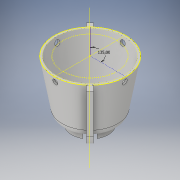
# Autodesk Inventor part: pot1
Saved by Autodesk Inventor 2019 (Build 230136000, 136)
## iProperties
Created: 2019-11-02
Part Number: pot1
Material: Generic
Document SubType Name: Modeling
Designer: assman
Density: 1 g/cm^3
Appearance: Default
Author: assman
## iProperties of the stored document pot1_3DPrint.ipt
Created: 2019-11-02
Part Number: pot1_3DPrint
Material: Generic
Document SubType Name: Modeling
Designer: assman
Density: 1 g/cm^3
Appearance: Default
Author: assman
Autodesk Inventor part; units mm, degrees
ref_plane "YZ Plane" through (0, 0, 0) normal (1, 0, 0) x (0, 1, 0)
ref_plane "XZ Plane" through (0, 0, 0) normal (0, 1, 0) x (-1, 0, 0)
ref_plane "XY Plane" through (0, 0, 0) normal (0, 0, 1) x (1, 0, 0)
sketch "Sketch2" plane through (0, 0, 0) normal (0, 0, 1) x (1, 0, 0)
  line L0 (0, 0) -> (28.321801, 0)
  line L1 (30.291416, 1.652704) -> (42.155372, 68.936543)
  arc A0 (28.321801, 0) -> (30.291416, 1.652704) centre (28.321801, 2) ccw
  line L2 (42.155372, 68.936543) -> (0, 68.936543)
  line L3 (0, 68.936543) -> (0, 0)
  point P0 (30, 0)
  dimension "d2" = 30
  dimension "d3" = 70
  dimension "d5" = 2
  constraints: 8 end point, 2 horizontal, 2 point on circle, 2 point on line, 2 tangent, 1 centre point, 1 perpendicular
  measures "d2" distance of L0.start point (30, 0)
  measures "d3" distance of point (30, 0) L1.end
  measures "d5" radius of A0
revolve "Revolution1" add sketch "Sketch2" angle 360 about axis through (0, 68.936543, 0) along (0, -1, 0)
sketch "Sketch3" plane through (0, 0, 0) normal (0, 0, 1) x (1, 0, 0)
  line L0 (42.155372, 68.936543) -> (30.291416, 1.652704)
  line L1 (-28.321801, 0) -> (28.321801, 0)
  arc A0 (28.321801, 0) -> (30.291416, 1.652704) centre (28.321801, 2) ccw
  line L2 (-28.321801, 0) -> (28.321801, 0)
  line L3 (33.488192, 70.4648) -> (21.624236, 3.180961)
  line L4 (0, -10) -> (28.321801, -10)
  line L5 (52.309639, 68.936543) -> (40.139494, -0.083778)
  arc A1 (28.321801, -10) -> (40.139494, -0.083778) centre (28.321801, 2) ccw
  line L6 (42.155372, 68.936543) -> (52.309639, 68.936543)
  line L7 (-42.155372, 68.936543) -> (42.155372, 68.936543)
  line L8 (0, 68.936543) -> (0, -10)
  line L9 (0, 68.936543) -> (42.155372, 68.936543)
  point P0 (0, 0)
  dimension "d7" = 10
  dimension "d8" = 10
  constraints: 14 end point, 3 parallel, 2 point on circle, 1 centre point, 1 collinear, 1 horizontal, 1 midpoint, 1 perpendicular, 1 tangent
  measures "d7" distance between parallel lines of L1 L4
  measures "d8" distance between parallel lines of L0 L5
revolve "Revolution2" add sketch "Sketch3" angle 360 about axis through (0, 68.936543, 0) along (0, -1, 0) separate body
combine bodies "Combine1" operation type subtract main body 2 bodies to subtract 1
sketch "Sketch5" plane through (0, 0, 0) normal (0, 0, 1) x (1, 0, 0)
  line L0 (0, 0) -> (28.321801, 0)
  arc A0 (28.321801, 0) -> (30.291416, 1.652704) centre (28.321801, 2) ccw
  line L1 (30.291416, 1.652704) -> (42.155372, 68.936543)
  line L2 (41.343031, 68.936543) -> (29.50357, 1.791622)
  arc A1 (28.321801, 0.8) -> (29.50357, 1.791622) centre (28.321801, 2) ccw
  line L3 (28.321801, 0.8) -> (0, 0.8)
  line L4 (42.155372, 68.936543) -> (41.343031, 68.936543)
  line L5 (-52.309639, 68.936543) -> (52.309639, 68.936543)
  line L6 (0, 0.8) -> (0, 0)
  line L7 (-40.139494, -0.083778) -> (40.139494, -0.083778)
  line L8 (0, -25.787309) -> (0, 84.723851)
  dimension "d10" = 0.8
  constraints: 8 end point, 2 point on circle, 1 centre point, 1 perpendicular, 1 point on line, 1 other
  measures "d10" distance between parallel lines of L1 L2
revolve "Revolution3" add sketch "Sketch5" angle 360 about axis through (0, -10, 0) along (0, 1, 0) separate body contours L6 L3 A1 L2 L4 L1 A0 L0
sketch "Sketch6" plane through (0, 0, 0) normal (0, 0, 1) x (1, 0, 0)
  line L0 (52.309639, 68.936543) -> (40.139494, -0.083778)
  arc A0 (28.321801, -10) -> (40.139494, -0.083778) centre (28.321801, 2) ccw
  line L1 (-28.321801, -10) -> (28.321801, -10)
  line L2 (0, -10) -> (28.321801, -10)
  arc A1 (28.321801, -11) -> (41.124302, -0.257426) centre (28.321801, 2) ccw
  line L3 (53.325065, 68.936543) -> (41.124302, -0.257426)
  line L4 (28.321801, -11) -> (0, -11)
  line L5 (0, -11) -> (0, -10)
  line L6 (52.309639, 68.936543) -> (53.325065, 68.936543)
  line L7 (0, -29.783146) -> (0, 85.389824)
  point P0 (0, 0)
  dimension "d13" = 1
  constraints: 10 end point, 4 point on circle, 2 centre point, 2 horizontal, 1 collinear, 1 midpoint, 1 parallel, 1 perpendicular
  measures "d13" distance between parallel lines of L0 L3
revolve "Revolution4" add sketch "Sketch6" angle 360 about axis through (0, -10, 0) along (0, 1, 0) separate body
sketch "Sketch7" plane through (0, 68.936543, 0) normal (0, 1, 0) x (1, 0, 0)
  circle A0 centre (0, 0) radius 41.343031 construction
  circle A1 centre (0, 0) radius 42.155372 construction
sketch "Sketch8" plane through (0, 0, 0) normal (1, 0, 0) x (0, 1, 0)
  circle A0 centre (60.936543, 0) radius 4
  line L0 (68.936543, 41.343031) -> (68.936543, -41.343031)
  point P0 (0, 0)
  dimension "d15" = 8
  dimension "d16" = 8
  constraints: 1 centre point
  measures "d15" diameter of A0
  measures "d16" distance from line of L0 A0.centre
extrude "Extrusion1" cut sketch "Sketch8" along normal mid plane 200 bodies 3
sketch "Sketch10" plane through (0, 68.936543, 0) normal (0, 1, 0) x (1, 0, 0)
  circle A0 centre (0, 0) radius 52.309639 construction
  line L0 (0, 52.309639) -> (0, -62.778673) construction
  constraints: 2 end point, 1 vertical, 1 vertical alignment, 1 other
ref_plane "Work Plane1" through (0, 68.936543, -52.309639) normal (-1, 0, 0) x (0, 0, 1)
ref_plane "Work Plane2" through (0, 68.936543, 0) normal (0, 0, 1) x (1, 0, 0)
sketch "Sketch11" plane through (0, 68.936543, 0) normal (0, 0, 1) x (1, 0, 0)
  circle A0 centre (0, -8) radius 4
  line L0 (-41.343031, 0) -> (41.343031, 0)
  point P0 (0, -68.936543)
  dimension "d20" = 8
  dimension "d21" = 8
  constraints: 1 centre point
  measures "d20" diameter of A0
  measures "d21" distance from line of L0 A0.centre
extrude "Extrusion2" cut sketch "Sketch11" along normal mid plane 200 bodies 3
thicken "Thicken1" operation add thickness 2 both sides no extend neighbours yes toward (0.5690288, -0.1736482, -0.803774) bodies 4 faces at (29.636646, 57.404215, -41.862847) (-7.864935, -4.931658, -38.525) (14.860047, -11, -5.989572)
sketch "Sketch12" plane through (0, 68.936543, 0) normal (0, 1, 0) x (1, 0, 0)
  line L0 (0, 0) -> (-39.142545, 39.142545)
  circle A0 centre (0, 0) radius 55.355918
  line L1 (0, 0) -> (55.355918, 0) construction
  dimension "d26" = 135
  constraints: 4 end point, 1 equal length, 1 horizontal, 2 other
  measures "d26" angle of L1 L0
ref_plane "Work Plane3" through (0, 68.936543, 0) normal (0.7071068, 0, -0.7071068) x (-0.7071068, 0, -0.7071068)
sketch "Sketch16" plane through (0, 0, 0) normal (0, 0, 1) x (1, 0, 0)
  circle A0 centre (0, 60.936543) radius 4
  line L0 (-52.309639, 68.936543) -> (52.309639, 68.936543)
  point P0 (0, 0)
  dimension "d29" = 8
  dimension "d30" = 8
  constraints: 1 centre point
  measures "d29" diameter of A0
  measures "d30" distance from line of L0 A0.centre
extrude "Extrusion3" cut sketch "Sketch16" along normal mid plane 200 bodies 4
sketch "Sketch17" plane through (0, 68.936543, 0) normal (0, 1, 0) x (1, 0, 0)
  circle A0 centre (0, 0) radius 55.355918 construction
  line L0 (0, 55.355918) -> (0, -55.355918) construction
  constraints: 2 end point, 2 point on circle, 1 vertical
sketch "Sketch18" plane through (0, 0, 0) normal (1, 0, 0) x (0, 1, 0)
  circle A0 centre (60.936543, 0) radius 4
  line L0 (68.936543, 52.309639) -> (68.936543, -52.309639)
  point P0 (0, 0)
  dimension "d33" = 8
  dimension "d34" = 8
  constraints: 1 centre point
  measures "d33" diameter of A0
  measures "d34" distance from line of L0 A0.centre
extrude "Extrusion4" cut sketch "Sketch18" along normal mid plane 200 bodies 4
sketch "Sketch19" plane through (0, 68.936543, 0) normal (0.7071068, 0, -0.7071068) x (-0.7071068, 0, -0.7071068)
  line L0 (-55.355918, 0) -> (-43.093917, -69.541265)
  line L1 (55.355918, 0) -> (43.093917, -69.541265)
  line L2 (65.203996, -1.736482) -> (52.941995, -71.277747)
  line L3 (-65.203996, -1.736482) -> (-52.941995, -71.277747)
  line L4 (-28.321801, -81.936543) -> (28.321801, -81.936543)
  arc A0 (28.321801, -81.936543) -> (43.093917, -69.541265) centre (28.321801, -66.936543) ccw
  arc A1 (-43.093917, -69.541265) -> (-28.321801, -81.936543) centre (-28.321801, -66.936543) ccw
  line L5 (-28.321801, -91.936543) -> (28.321801, -91.936543)
  arc A2 (-52.941995, -71.277747) -> (-28.321801, -91.936543) centre (-28.321801, -66.936543) ccw
  arc A3 (28.321801, -91.936543) -> (52.941995, -71.277747) centre (28.321801, -66.936543) ccw
  line L6 (65.203996, -1.736482) -> (55.355918, 0)
  line L7 (-65.203996, -1.736482) -> (-55.355918, 0)
  circle A4 centre (59.072995, -7.713262) radius 3
  circle A5 centre (52.166428, -46.882352) radius 3
  circle A6 centre (40.908295, -81.936543) radius 3
  line L8 (0, -92.777343) -> (0, -9.509843)
  line L9 (0, -9.509843) -> (0, -97.349981)
  circle A7 centre (-59.072995, -7.713262) radius 3
  circle A8 centre (-52.166428, -46.882352) radius 3
  circle A9 centre (-40.908295, -81.936543) radius 3
  circle A10 centre (0, -87.421042) radius 3
  point P0 (0, -68.936543)
  dimension "d37" = 10
  dimension "d38" = 10
  dimension "d39" = 10
  dimension "d40" = 10
  dimension "d41" = 10
  dimension "d42" = 6
  dimension "d43" = 6
  dimension "d44" = 6
  dimension "d45" = 6
  constraints: 14 end point, 11 centre point, 8 point on circle, 3 parallel, 3 symmetric about line, 2 point on line, 1 perpendicular, 1 vertical, 3 other
  measures "d37" distance between parallel lines of L1 L2
  measures "d38" distance between parallel lines of L0 L3
  measures "d39" distance between parallel lines of L4 L5
  measures "d40" radial gap between concentric circles of A1 A2
  measures "d41" radial gap between concentric circles of A0 A3
  measures "d42" diameter of A4
  measures "d43" diameter of A5
  measures "d44" diameter of A6
  measures "d45" diameter of A10
extrude "Extrusion5" add sketch "Sketch19" along normal mid plane 8 contours L0 A1 L4 L8 A10 L5 A2 L3 L7 | L4 A0 L1 L6 L2 A3 L5 L8 A10 bodies 4
sketch "Sketch20" plane through (0, -13, 0) normal (0, -1, 0) x (0.7071068, 0, -0.7071068)
  line L0 (-4, -28.03791) -> (-4, 28.03791) construction
  arc A0 (-8, 27.168445) -> (-8, -27.168445) centre (0, 0) ccw
  line L1 (4, 28.03791) -> (4, -28.03791) construction
  arc A1 (4, -28.03791) -> (4, 28.03791) centre (0, 0) ccw construction
  line L2 (-8, 22.968456) -> (-8, -22.968456) construction
  arc A2 (-8, 22.968456) -> (-8, -22.968456) centre (0, 0) ccw
  line L3 (8, -22.968456) -> (8, 22.968456) construction
  arc A3 (8, -22.968456) -> (8, 22.968456) centre (0, 0) ccw
  line L4 (8, -22.968456) -> (8, -27.168445)
  line L5 (8, 22.968456) -> (8, 27.168445)
  circle A4 centre (0, 0) radius 28.321801 construction
  line L6 (-8, 22.968456) -> (-8, 27.168445)
  line L7 (-8, -22.968456) -> (-8, -27.168445)
  arc A5 (8, -27.168445) -> (8, 27.168445) centre (0, 0) ccw
  dimension "d10" = 0.8
  dimension "d48" = 4
  dimension "d49" = 4
  constraints: 12 end point, 8 point on circle, 4 centre point, 2 vertical, 1 parallel, 1 point on line, 5 other
  measures "d48" radial gap between concentric circles of A0 A2
  measures "d49" radial gap between concentric circles of A1 A3
extrude "Extrusion6" add sketch "Sketch20" along normal up to surface (10 mm away) bodies 4
split body "Split1" result two bodies by plane through (0, 68.936543, 0) normal (0.7071068, 0, -0.7071068) bodies 4 first body at (-31.324656, 34.252734, -37.331271)
body "Solid2"
body "Solid3"
body "Solid5"
body "Solid6"
